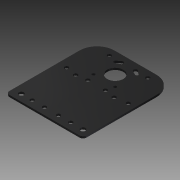
# Autodesk Inventor part: x_motor_mount_v2
Saved by Autodesk Inventor 2014 (Build 180170000, 170)
## iProperties
Created: 2013-07-17
Part Number: x_motor_mount_v2
Material: Steel, Mild
Document SubType Name: Modeling
Designer: Edward
Density: 7.86 g/cm^3
Appearance: Lacquer - Black
d0: 110.000 mm
d1: 130.000 mm
d2: 65.000 mm
d3: 55.000 mm
d4: 2.657 mm
d5: 0.00 deg
d15: 7.140 mm
d16: 5.500 mm
d17: 64.600 mm
d18: 10.000 mm
d19: 12.000 mm
d21: 12.000 mm
d23: 0.00 deg
d24: 2.000 ul
d26: 88.000 mm
d27: 23.000 mm
d28: 29.000 mm
d29: 4.000 mm
d30: 15.500 mm
d31: 15.500 mm
d36: 55.000 mm
d38: 0.00 deg
d39: 25.000 mm
d41: 5.500 mm
d42: 74.500 mm
d43: 42.500 mm
d45: 0.00 deg
d49: 2.000 ul
d51: 31.000 mm
d52: 2.000 ul
d54: 31.000 mm
Author: Edward
Autodesk Inventor part; units mm, degrees
ref_plane "YZ Plane" through (0, 0, 0) normal (1, 0, 0) x (0, 1, 0)
ref_plane "XZ Plane" through (0, 0, 0) normal (0, 1, 0) x (-1, 0, 0)
ref_plane "XY Plane" through (0, 0, 0) normal (0, 0, 1) x (1, 0, 0)
sketch "Sketch1" plane through (0, 0, 0) normal (0, 0, 1) x (1, 0, 0)
  line L0 (-55, 65) -> (55, 65)
  line L1 (55, 65) -> (55, -65)
  line L2 (55, -65) -> (-55, -65)
  line L3 (-55, -65) -> (-55, 65)
  point P0 (0, 0)
  dimension "d0" = 110
  dimension "d1" = 130
  dimension "d2" = 65
  dimension "d3" = 55
  constraints: 8 end point, 2 parallel, 1 horizontal, 1 perpendicular
  measures "d0" distance of L1.end L2.end
  measures "d1" distance of L0.end L1.end
  measures "d2" distance from line of L0 point (0, 0)
  measures "d3" distance from line of L3 point (0, 0)
extrude "profile" add sketch "Sketch1" along normal blind 2.6568
sketch "Sketch3" plane through (0, 0, 2.6568) normal (0, 0, 1) x (1, 0, 0)
  line L0 (-55, 65) -> (-55, -65) projected
  line L1 (-55, -65) -> (55, -65) projected
  circle A0 centre (-43, -55) radius 3.57
  circle A1 centre (-43, 9.6) radius 2.75
  circle A2 centre (-43, 9.6) radius 11.75 construction
  point P0 (0, 0)
  dimension "d15" = 7.14
  dimension "d16" = 5.5
  dimension "d17" = 64.6
  dimension "d18" = 10
  dimension "d19" = 12
  dimension "d21" = 12
  constraints: 3 centre point, 1 coincident
  measures "d15" diameter of A0
  measures "d16" diameter of A1
  measures "d17" distance of A0.centre A1.centre
  measures "d18" distance from line of L1 A0.centre
  measures "d19" distance from line of L0 A0.centre
  measures "d21" distance from line of L0 A2.centre
extrude "Extrusion3" cut sketch "Sketch3" against normal through all
pattern_linear "Rectangular Pattern2" count 2 spacing 88 along (1, 0, 0) of "Extrusion3"
sketch "Sketch4" plane through (0, 0, 2.6568) normal (0, 0, 1) x (1, 0, 0)
  line L0 (55, 65) -> (-55, 65) projected
  line L1 (55, -65) -> (55, 65) projected
  circle A0 centre (0, 36) radius 11.5
  circle A1 centre (-15.5, 51.5) radius 2
  circle A2 centre (15.5, 51.5) radius 2
  circle A3 centre (-15.5, 20.5) radius 2
  circle A4 centre (15.5, 20.5) radius 2
  point P0 (0, 0)
  dimension "d27" = 23
  dimension "d28" = 29
  dimension "d29" = 4
  dimension "d30" = 15.5
  dimension "d31" = 15.5
  dimension "d36" = 55
  dimension "d51" = 31
  dimension "d54" = 31
  constraints: 5 centre point, 1 horizontal, 1 vertical, 6 other
  measures "d27" diameter of A0
  measures "d28" distance from line of L0 A0.centre
  measures "d29" diameter of A1
  measures "d30" horizontal distance of A0.centre A1.centre
  measures "d31" horizontal distance of A1.centre A0.centre
  measures "d36" distance from line of L1 A0.centre
  measures "d51" distance of A1.centre A2.centre
  measures "d54" distance of A1.centre A3.centre
extrude "nema17_mount" cut sketch "Sketch4" against normal through all
fillet "Fillet1" radius 25 2 edges at (55, 65, 1.3284) (-55, 65, 1.3284)
sketch "Sketch5" plane through (0, 0, 2.6568) normal (0, 0, 1) x (1, 0, 0)
  line L0 (-55, 65) -> (-55, -65) projected
  line L1 (-55, -65) -> (55, -65) projected
  circle A0 centre (-12.5, 9.5) radius 2.75
  line L2 (30, 65) -> (-30, 65) projected
  circle A1 centre (12.5, 9.5) radius 2.75
  point P0 (67.5, -65)
  point P1 (-72.5, 60)
  point P2 (-72.5, -60)
  point P3 (-67.5, -65)
  point P4 (0, 0)
  dimension "d41" = 5.5
  dimension "d42" = 74.5
  dimension "d43" = 42.5
  dimension "d59" = 25
  constraints: 2 centre point, 1 horizontal, 3 other
  measures "d41" diameter of A0
  measures "d42" distance from line of L1 A0.centre
  measures "d59" distance of A0.centre A1.centre
extrude "idler_holes" cut sketch "Sketch5" against normal through all
sketch "Sketch7" plane through (0, 0, 2.6568) normal (0, 0, 1) x (1, 0, 0)
  circle A0 centre (-15.5, 51.5) radius 2 projected
  line L0 (-55, 40) -> (-55, -65) projected
  line L1 (30, 65) -> (-30, 65) projected
  arc A1 (-9.3427, 52.3297) -> (-11.7335, 57.1348) centre (-10, 55) ccw
  arc A2 (11.7395, 57.13) -> (8.8336, 52.5096) centre (10, 55) ccw
  line L2 (-11.7335, 57.1348) -> (-16.7607, 53.0526)
  line L3 (-8.2665, 52.8652) -> (-14.6091, 49.7094)
  circle A3 centre (15.5, 51.5) radius 2 projected
  line L4 (8.8336, 52.5096) -> (14.6274, 49.7004)
  line L5 (16.9616, 52.8652) -> (11.7395, 57.13)
  point P0 (0, 0)
  dimension "d70" = 5.5
  dimension "d71" = 5.5
  dimension "d72" = 10
  dimension "d73" = 10
  dimension "d74" = 20
  dimension "d75" = 45
  constraints: 10 point on circle, 8 end point, 5 tangent, 2 centre point, 2 point on line
  measures "d70" diameter of A1
  measures "d71" diameter of A2
  measures "d72" distance from line of L1 A2.centre
  measures "d73" distance from line of L1 A1.centre
  measures "d74" distance of A2.centre A1.centre
  measures "d75" distance from line of L0 A1.centre
extrude "Extrusion7" cut sketch "Sketch7" against normal through all contours A0 L2 A1 L3 | L5 A3 L4 A2 | L5 A3 picked at (16.0496, 50.6933)
sketch "Sketch8" plane through (0, 0, 2.6568) normal (0, 0, 1) x (1, 0, 0)
  line L0 (-55, 40) -> (-55, -65) projected
  line L1 (-55, -65) -> (55, -65) projected
  circle A0 centre (-10, -55) radius 2.75
  circle A1 centre (10, -55) radius 2.75
  point P0 (0, 0)
  dimension "d78" = 5.5
  dimension "d79" = 5.5
  dimension "d80" = 20
  dimension "d81" = 10
  dimension "d82" = 10
  dimension "d83" = 45
  constraints: 2 centre point
  measures "d78" diameter of A0
  measures "d79" diameter of A1
  measures "d80" distance of A0.centre A1.centre
  measures "d81" distance from line of L1 A0.centre
  measures "d82" distance from line of L1 A1.centre
  measures "d83" distance from line of L0 A0.centre
extrude "Extrusion8" cut sketch "Sketch8" against normal through all
sketch "Sketch9" plane through (0, 0, 2.6568) normal (0, 0, 1) x (1, 0, 0)
  line L0 (-55, 40) -> (-55, -65) projected
  line L1 (-55, -65) -> (55, -65) projected
  circle A0 centre (-27.5, 7) radius 2.75
  point P0 (0, 0)
  dimension "d86" = 5.5
  dimension "d87" = 27.5
  dimension "d88" = 72
  constraints: 1 centre point
  measures "d86" diameter of A0
  measures "d87" distance from line of L0 A0.centre
  measures "d88" distance from line of L1 A0.centre
extrude "Extrusion9" cut sketch "Sketch9" against normal through all
pattern_linear "Rectangular Pattern4" count 2 spacing 55 along (1, 0, 0) count 2 spacing 62 along (0, -1, 0) of "Extrusion9"
fillet "Fillet3" radius 5 2 edges at (55, -65, 1.3284) (-55, -65, 1.3284)
sketch "Sketch10" plane through (0, 0, 2.6568) normal (0, 0, 1) x (1, 0, 0)
  line L0 (30, 65) -> (-30, 65) projected
  line L1 (-55, 40) -> (-55, -60) projected
  circle A0 centre (-27.5, 55) radius 2.75
  circle A1 centre (27.5, 55) radius 2.75
  point P0 (0, 0)
  dimension "d98" = 5.5
  dimension "d99" = 5.5
  dimension "d100" = 27.5
  dimension "d101" = 82.5
  dimension "d102" = 10
  dimension "d103" = 10
  constraints: 2 centre point
  measures "d98" diameter of A0
  measures "d99" diameter of A1
  measures "d100" distance from line of L1 A0.centre
  measures "d101" distance from line of L1 A1.centre
  measures "d102" distance from line of L0 A0.centre
  measures "d103" distance from line of L0 A1.centre
extrude "Extrusion10" cut sketch "Sketch10" against normal through all
equation "\"d2\" = 0.5 * d1"
equation "\"d3\" = 0.5 * d0"
equation "\"d72\" = d73"
equation "\"d82\" = d81"
body "Solid1"
